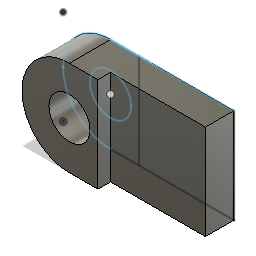
LCD Clamp v4 (Autodesk Fusion 360 design; units mm, degrees)
Autodesk Fusion 360 part; units mm, degrees
sketch "Sketch1" plane through (0, 0, 0) normal (0, 0, 1) x (1, 0, 0)
  line L0 (3.81, 0) -> (13.716, 0)
  line L1 (13.716, 0) -> (13.716, 7.62)
  line L2 (13.716, 7.62) -> (3.81, 7.62)
  line L3 (0, 3.81) -> (0, 3.81)
  line L4 (6.096, 7.62) -> (6.096, 0)
  circle A0 centre (3.81, 3.81) radius 1.651
  arc A1 (0, 3.81) -> (3.81, 0) centre (3.81, 3.81) ccw
  arc A2 (3.81, 7.62) -> (0, 3.81) centre (3.81, 3.81) ccw
  point P0 (0, 7.62)
  dimension "d1" = 7.62
  dimension "d2" = 13.716
  dimension "d3" = 7.62
  dimension "d4" = 3.302
  dimension "d6" = 3.81
  dimension "d7" = 3.81
  dimension "d8" = 3.81
  constraint horizontal L0
  constraint vertical L1
  constraint horizontal L2
  constraint coincident L2 L4.start
  constraint coincident L0 L4.end
  constraint perpendicular L0 L4
  constraint coincident origin L0
  constraint tangent L0 A1
  constraint coincident P0 L2
  constraint coincident P0 L3
  constraint tangent L2 A2
  measures "d1" distance of origin P0
  measures "d2" distance of origin L0.end
  measures "d3" distance of L1 L4
  measures "d4" diameter of A0
  measures "d6" distance of L2 A0.centre
  measures "d7" radius of A1
  measures "d8" radius of A2
extrude "Extrude1" add sketch "Sketch1" along normal blind 3.302 contours L0 L2 L4 A1 A2
extrude "Extrude2" add sketch "Sketch1" along normal blind 2.286 contours L0 L1 L2 L4
